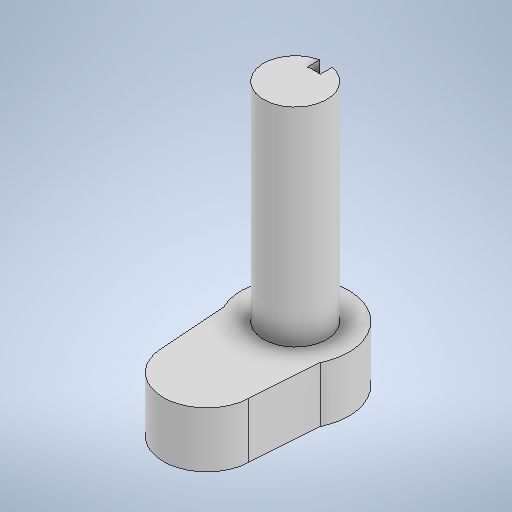
# Autodesk Inventor part: Servo_Shaft_V2
Saved by Autodesk Inventor 2025.3 (Build 293356000, 356)
## iProperties
Created: 2026-04-10
Part Number: Servo_Shaft_V2
Material: Generic
Document SubType Name: Modeling
Designer: kamal
Density: 1 g/cm^3
Appearance: Default
Mass: 5.65431 g
Surface Area: 27.7969 cm^2
Volume: 5.65431 cm^3
Author: kamal
Autodesk Inventor part; units mm, degrees
ref_plane "YZ Plane" through (0, 0, 0) normal (1, 0, 0) x (0, 1, 0)
ref_plane "XZ Plane" through (0, 0, 0) normal (0, 1, 0) x (-1, 0, 0)
ref_plane "XY Plane" through (0, 0, 0) normal (0, 0, 1) x (1, 0, 0)
sketch "Sketch1" plane through (0, 0, 0) normal (0, 1, 0) x (-1, 0, 0)
  arc A0 (-2.75, 2.1651) -> (2.75, 2.1651) centre (0, 0) ccw
  line L0 (-1.9, 14.1) -> (-2.75, 2.1651)
  line L1 (1.8987, 14.0987) -> (2.75, 2.1651)
  arc A1 (1.8987, 14.0987) -> (-1.9, 14.1) centre (-0.0007, 14.05) ccw
  circle A2 centre (0, 0) radius 0.5
  arc A3 (-7.6535, 3.6978) -> (7.6533, 3.6982) centre (0, 0) ccw
  line L2 (-7.6535, 3.6978) -> (-6.8928, 14.3783)
  arc A4 (6.8916, 14.3762) -> (-6.8928, 14.3783) centre (-0.0007, 14.05) ccw
  line L3 (6.8916, 14.3762) -> (7.6533, 3.6982)
  point P0 (0, 15.95)
  dimension "d0" = 1
  dimension "d9" = 1.9
  dimension "d10" = 15.95
  dimension "d11" = 3.5
  dimension "d17" = 5
  constraints: 9 point on circle, 8 end point, 5 centre point, 1 coincident, 1 concentric, 3 other
  measures "d0" diameter of A2
  measures "d9" radius of A1
  measures "d10" distance of point (0, 0) point (0, 15.95)
  measures "d11" radius of A0
  measures "d17" distance between parallel lines of L1 L3
extrude "Extrusion1" add sketch "Sketch1" along normal blind 3.8 contours L2 A4 L3 A3
sketch "Sketch2" plane through (0, 3.8, 0) normal (0, 1, 0) x (1, 0, 0)
  arc A0 (2.75, -2.1651) -> (-2.75, -2.1651) centre (0, 0) ccw projected
  circle A1 centre (0, 0) radius 3.5
  arc A2 (-6.8916, -14.3762) -> (6.8928, -14.3783) centre (0.0007, -14.05) ccw projected
  line L0 (-7.6533, -3.6982) -> (-6.8916, -14.3762) projected
  arc A3 (7.6535, -3.6978) -> (-7.6533, -3.6982) centre (0, 0) ccw projected
  line L1 (6.8928, -14.3783) -> (7.6535, -3.6978) projected
  arc A4 (2.75, -2.1651) -> (-2.75, -2.1651) centre (0, 0) ccw projected
  point P0 (2.75, -2.1651)
  point P1 (-2.75, -2.1651)
  constraints: 1 centre point, 1 coincident, 1 concentric
extrude "Extrusion2" add sketch "Sketch2" along normal blind 5
sketch "Sketch3" plane through (0, 8.8, 0) normal (0, 1, 0) x (1, 0, 0)
  arc A0 (2.75, -2.1651) -> (-2.75, -2.1651) centre (0, 0) ccw projected
  circle A1 centre (0, 0) radius 5
  dimension "d22" = 10
  constraints: 1 centre point, 1 coincident
  measures "d22" diameter of A1
extrude "Extrusion3" add sketch "Sketch3" along normal blind 8
sketch "Sketch4" plane through (0, 16.8, 0) normal (0, 1, 0) x (1, 0, 0)
  circle A0 centre (0, 0) radius 5
  line L0 (1, 3) -> (-1, 3)
  line L1 (-1, 3) -> (-1, 7)
  line L2 (-1, 7) -> (1, 7)
  line L3 (1, 7) -> (1, 3)
  line L4 (1, 3) -> (-1, 7) construction
  line L5 (-1, 3) -> (1, 7) construction
  point P0 (0, 5)
  point P1 (-1, 4.899)
  point P2 (1, 4.899)
  dimension "d25" = 10
  dimension "d26" = 2
  dimension "d27" = 4
  dimension "d28" = 1
  constraints: 12 end point, 2 midpoint, 2 parallel, 1 coincident, 1 horizontal, 1 perpendicular, 3 other
  measures "d26" distance of L1.end L2.end
  measures "d27" distance of L0.end L1.end
  measures "d28" distance from line of point (0, 0) L3
extrude "Extrusion4" add sketch "Sketch4" along normal blind 25 contours A0 L1 L0 L3 picked at (-0.1517, 0.3403)
sketch "Sketch5" plane through (0, 3.8, 0) normal (0, -1, 0) x (1, 0, 0)
  circle A0 centre (0, 0) radius 3.5
  dimension "d31" = 7
  constraints: 1 centre point, 1 coincident
  measures "d31" diameter of A0
extrude "Extrusion5" add sketch "Sketch5" against normal blind 5
body "Solid1"
